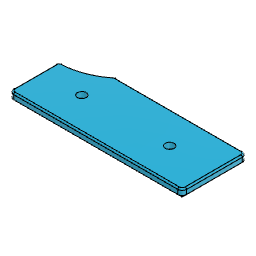
couvercle_connecteur_moteur_KOSMOS3-0 (Autodesk Fusion 360 design; units mm, degrees)
Autodesk Fusion 360 part; units mm, degrees
sketch "Esquisse1" plane through (0, 0, 0) normal (0, 0, 1) x (1, 0, 0)
  line L0 (0, 0) -> (59, 0)
  line L1 (59, 0) -> (59, 22)
  line L2 (59, 22) -> (0, 22)
  line L3 (0, 22) -> (0, 0)
  line L4 (0, 0) -> (0, 17) construction
  line L5 (0, 17) -> (0, 39) construction
  arc A0 (0, 17) -> (13.9642, 22) centre (0, 39) ccw
  dimension "d1" = 22
  dimension "d2" = 59
  dimension "d3" = 17
  dimension "d4" = 22
  constraint horizontal L0
  constraint vertical L1
  constraint horizontal L2
  constraint vertical L3
  constraint coincident L0.start L3.end
  constraint perpendicular L0 L4
  constraint perpendicular L2 L5
  constraint coincident L5.end A0.centre
  constraint coincident L2 A0.end
  measures "d1" distance of L0.start L2.end
  measures "d2" distance of L0.start L0.end
  measures "d3" distance of L0.start L4.end
  measures "d4" distance of L4.end L5.end
extrude "Extrusion1" add sketch "Esquisse1" along normal blind 2 contours L0 L1 L2 L3 A0
sketch "Esquisse2" plane through (0, 0, 2) normal (0, 0, 1) x (-1, 0, 0)
  line L0 (0, 0) -> (-59, 0)
  line L1 (-59, 0) -> (-59, -22)
  line L2 (-59, -22) -> (-13.9642, -22)
  arc A0 (0, -17) -> (-13.9642, -22) centre (0, -39) ccw
  line L3 (0, -17) -> (0, 0)
  arc A1 (-1.4, -15.6419) -> (-14.4568, -20.6) centre (0, -39) ccw
  line L4 (-57.6, -20.6) -> (-14.4568, -20.6)
  line L5 (-57.6, -1.4) -> (-57.6, -20.6)
  line L6 (-1.4, -1.4) -> (-57.6, -1.4)
  line L7 (-1.4, -15.6419) -> (-1.4, -1.4)
  dimension "d7" = -1.4
extrude "Extrusion11" add sketch "Esquisse2" against normal blind 3.7 contours A1 L4 L5 L6 L7
chamfer "Chanfrein3" distance 0.3 angle 45 5 edges at (29.5, 1.4, -1.7) (1.4, 8.521, -1.7) (8.307, 17.1241, -1.7) (36.0284, 20.6, -1.7) (57.6, 11, -1.7)
fillet "Congé7" radius 1.5 3 edges at (0, 0, 1) (59, 0, 1) (59, 22, 1)
fillet "Congé8" radius 1 2 edges at (13.9642, 22, 1) (0, 17, 1)
fillet "Congé9" radius 0.5 10 edges at (0.4393, 0.4393, 2) (29.5, 0, 2) (58.5607, 0.4393, 2) (59, 11, 2) (58.5607, 21.5607, 2) (35.9089, 22, 2) (13.9881, 21.9441, 2) (7.7031, 18.3927, 2) (0.2777, 16.7133, 2) (0, 8.7609, 2)
hole "Perçage1" at (43.74, 11, 2) direction (0, 0, -1) diameter 1.5 depth 9 tip angle 180 counterbore diameter 3 counterbore depth 2
pattern_linear "Réseau R1" count 2 spacing 30 along (-1, 0, 0) of "Perçage1"
equation "d5 = 2 mm"
equation "d76 = d5"
